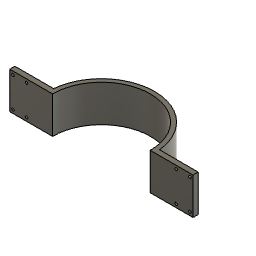
ClampMnt v4 (Autodesk Fusion 360 design; units mm, degrees)
Autodesk Fusion 360 part; units mm, degrees
sketch "Sketch1" plane through (0, 0, 0) normal (0, 1, 0) x (1, 0, 0)
  line L0 (0, 57.15) -> (0, 62.15)
  line L1 (57.15, 0) -> (107.15, 0)
  line L2 (107.15, 0) -> (107.15, 6)
  line L3 (107.15, 6) -> (61.8597, 6)
  arc A0 (57.15, 0) -> (0, 57.15) centre (0, 0) ccw
  arc A1 (61.8597, 6) -> (0, 62.15) centre (0, 0) ccw
  constraint coincident A0.centre A1.centre
  constraint coincident A0.centre L0
sketch "Sketch7" plane through (0, 0, 0) normal (0, 1, 0) x (1, 0, 0)
extrude "Extrude8" add sketch "Sketch1" along normal blind 43 makes body 1
sketch "Sketch8" plane through (0, 0, -6) normal (0, 0, -1) x (-1, 0, 0)
  line L0 (-107.15, 0) -> (-61.8597, 0)
  line L1 (-61.8597, 0) -> (-61.8597, 43)
  line L2 (-61.8597, 43) -> (-107.15, 43)
  line L3 (-107.15, 43) -> (-107.15, 0)
  circle A0 centre (-103.4242, 4) radius 1.5
  circle A1 centre (-103.4242, 39) radius 1.5
  circle A2 centre (-87.4242, 4) radius 1.5
  circle A3 centre (-87.4242, 39) radius 1.5
  dimension "d26" = 3
  dimension "d27" = 3
  dimension "d28" = 16
  dimension "d29" = 3
  dimension "d30" = 3
  measures "d26" diameter of A0
  measures "d27" diameter of A1
  measures "d28" distance of A0.centre A2.centre
  measures "d29" diameter of A2
  measures "d30" diameter of A3
extrude "Extrude9" cut sketch "Sketch8" against normal blind 18 contours A0 | A1 | A2 | A3 bodies 1
mirror "Mirror1" about plane through (0, 0, 0) normal (1, 0, 0) of bodies 1 makes body 2
combine "Combine1" operation add target body 1 tool bodies 2
